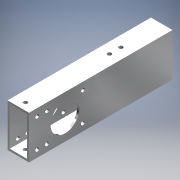
# Autodesk Inventor part: SupportExtrusion
Saved by Autodesk Inventor 2019.4 (Build 234330000, 330)
## iProperties
Created: 2019-12-31
Part Number: SupportExtrusion
Material: Aluminum 6061
Document SubType Name: Modeling
Designer: Mark
Mass: 206.469 g
Surface Area: 554.94 cm^2
Volume: 76.4699 cm^3
Density: 2.7 g/cm^3
Appearance: Aluminum - Flat
Author: Mark
Autodesk Inventor part; units mm, degrees
ref_plane "YZ Plane" through (0, 0, 0) normal (1, 0, 0) x (0, 1, 0)
ref_plane "XZ Plane" through (0, 0, 0) normal (0, 1, 0) x (-1, 0, 0)
ref_plane "XY Plane" through (0, 0, 0) normal (0, 0, 1) x (1, 0, 0)
sketch "Sketch1" plane through (0, 0, 0) normal (0, 0, 1) x (1, 0, 0)
  line L0 (-15, -30) -> (15, -30)
  line L1 (15, -30) -> (15, 30)
  line L2 (15, 30) -> (-15, 30)
  line L3 (-15, 30) -> (-15, -30)
  line L4 (-15, -30) -> (15, 30) construction
  line L5 (15, -30) -> (-15, 30) construction
  line L6 (-12, -27) -> (12, -27)
  line L7 (12, -27) -> (12, 27)
  line L8 (12, 27) -> (-12, 27)
  line L9 (-12, 27) -> (-12, -27)
  line L10 (-12, -27) -> (12, 27) construction
  line L11 (12, -27) -> (-12, 27) construction
  point P0 (0, 0)
  dimension "d0" = 30
  dimension "d1" = 60
  dimension "d2" = 24
  dimension "d3" = 54
  constraints: 24 end point, 4 midpoint, 4 parallel, 2 horizontal, 2 perpendicular
  measures "d0" distance of L2.end L1.end
  measures "d1" distance of L1.end L0.end
  measures "d2" distance of L8.end L7.end
  measures "d3" distance of L7.end L6.end
extrude "Extrusion1" add sketch "Sketch1" along normal blind 200
sketch "Sketch2" plane through (-15, -30, 0) normal (-1, 0, 0) x (0, 0, 1)
  circle A0 centre (188.5, 50) radius 2.75
  circle A1 centre (188.5, 10) radius 2.75
  line L0 (200, 60) -> (200, 0) projected
  line L1 (0, 0) -> (200, 0) projected
  line L2 (0, 60) -> (200, 60) projected
  point P0 (0, 30)
  dimension "d6" = 5.5
  dimension "d7" = 5.5
  dimension "d8" = 11.5
  dimension "d9" = 10
  dimension "d10" = 11.5
  dimension "d11" = 10
  constraints: 2 centre point
  measures "d6" diameter of A0
  measures "d7" diameter of A1
  measures "d8" distance from line of L0 A1.centre
  measures "d9" distance from line of L1 A1.centre
  measures "d10" distance from line of L0 A0.centre
  measures "d11" distance from line of L2 A0.centre
extrude "Extrusion2" cut sketch "Sketch2" against normal blind 30
sketch "Sketch3" plane through (-15, 30, 0) normal (0, 1, 0) x (1, 0, 0)
  circle A0 centre (15, -73) radius 2.75
  circle A1 centre (15, -57) radius 2.75
  line L0 (0, 0) -> (0, -200) projected
  line L1 (30, -200) -> (0, -200) projected
  circle A2 centre (15, -190) radius 2.75
  line L2 (30, 0) -> (30, -200) projected
  point P0 (15, 0)
  dimension "d14" = 5.5
  dimension "d15" = 5.5
  dimension "d16" = 15
  dimension "d17" = 15
  dimension "d18" = 127
  dimension "d19" = 16
  dimension "d40" = 5.5
  dimension "d41" = 10
  dimension "d42" = 15
  constraints: 3 centre point
  measures "d14" diameter of A0
  measures "d15" diameter of A1
  measures "d16" distance from line of L0 A1.centre
  measures "d17" distance from line of L0 A0.centre
  measures "d18" distance from line of L1 A0.centre
  measures "d19" distance of A0.centre A1.centre
  measures "d40" diameter of A2
  measures "d41" distance from line of L1 A2.centre
  measures "d42" distance from line of L2 A2.centre
extrude "Extrusion3" cut sketch "Sketch3" against normal blind 60
sketch "Sketch4" plane through (-15, -30, 0) normal (-1, 0, 0) x (0, 0, 1)
  circle A0 centre (150, 30) radius 20
  line L0 (125, 50) -> (175, 50)
  line L1 (175, 50) -> (175, 10)
  line L2 (175, 10) -> (125, 10)
  line L3 (125, 10) -> (125, 50)
  line L4 (125, 50) -> (175, 10) construction
  line L5 (175, 50) -> (125, 10) construction
  circle A1 centre (175, 50) radius 2.75
  circle A2 centre (175, 10) radius 2.75
  circle A3 centre (125, 10) radius 2.75
  circle A4 centre (125, 50) radius 2.75
  line L6 (200, 60) -> (200, 0) projected
  line L7 (0, 0) -> (200, 0) projected
  circle A5 centre (75, 50) radius 2.75
  circle A6 centre (100, 30) radius 20
  circle A7 centre (125, 50) radius 2.75
  circle A8 centre (125, 10) radius 2.75
  circle A9 centre (75, 10) radius 2.75
  circle A10 centre (25, 50) radius 2.75
  circle A11 centre (50, 30) radius 20
  circle A12 centre (75, 50) radius 2.75
  circle A13 centre (75, 10) radius 2.75
  circle A14 centre (25, 10) radius 2.75
  circle A15 centre (-25, 50) radius 2.75
  circle A16 centre (0, 30) radius 20
  circle A17 centre (25, 50) radius 2.75
  circle A18 centre (25, 10) radius 2.75
  circle A19 centre (-25, 10) radius 2.75
  circle A20 centre (-75, 50) radius 2.75
  circle A21 centre (-50, 30) radius 20
  circle A22 centre (-25, 50) radius 2.75
  circle A23 centre (-25, 10) radius 2.75
  circle A24 centre (-75, 10) radius 2.75
  circle A25 centre (-125, 50) radius 2.75
  circle A26 centre (-100, 30) radius 20
  circle A27 centre (-75, 50) radius 2.75
  circle A28 centre (-75, 10) radius 2.75
  circle A29 centre (-125, 10) radius 2.75
  circle A30 centre (-175, 50) radius 2.75
  circle A31 centre (-150, 30) radius 20
  circle A32 centre (-125, 50) radius 2.75
  circle A33 centre (-125, 10) radius 2.75
  circle A34 centre (-175, 10) radius 2.75
  circle A35 centre (-225, 50) radius 2.75
  circle A36 centre (-200, 30) radius 20
  circle A37 centre (-175, 50) radius 2.75
  circle A38 centre (-175, 10) radius 2.75
  circle A39 centre (-225, 10) radius 2.75
  circle A40 centre (-275, 50) radius 2.75
  circle A41 centre (-250, 30) radius 20
  circle A42 centre (-225, 50) radius 2.75
  circle A43 centre (-225, 10) radius 2.75
  circle A44 centre (-275, 10) radius 2.75
  circle A45 centre (-325, 50) radius 2.75
  circle A46 centre (-300, 30) radius 20
  circle A47 centre (-275, 50) radius 2.75
  circle A48 centre (-275, 10) radius 2.75
  circle A49 centre (-325, 10) radius 2.75
  point P0 (0, 30)
  dimension "d22" = 40
  dimension "d23" = 50
  dimension "d24" = 40
  dimension "d25" = 5.5
  dimension "d26" = 5.5
  dimension "d27" = 5.5
  dimension "d28" = 5.5
  dimension "d29" = 50
  dimension "d30" = 10
  dimension "d33" = 50
  constraints: 50 centre point, 12 end point, 4 coincident, 2 horizontal, 2 midpoint, 2 parallel, 1 perpendicular, 90 other
  measures "d22" diameter of A0
  measures "d23" distance of L1.end L2.end
  measures "d24" distance of L0.end L1.end
  measures "d25" diameter of A1
  measures "d26" diameter of A2
  measures "d27" diameter of A3
  measures "d28" diameter of A4
  measures "d29" distance from line of L6 A0.centre
  measures "d30" distance between parallel lines of L7 L2
  measures "d33" distance of A4.centre A5.centre
extrude "Extrusion4" cut sketch "Sketch4" against normal blind 60 contours A0 | A4 L3 L0 | L0 L3 A4 | A1 L1 L0 | L0 L1 A1 | A2 L1 L2 | L2 L1 A2 | A3 L3 L2 | L2 L3 A3
sketch "Sketch5" plane through (-15, -30, 0) normal (-1, 0, 0) x (0, 0, 1)
  circle A0 centre (38.5, 50) radius 2.75
  circle A1 centre (91.5, 50) radius 2.75
  circle A2 centre (91.5, 10) radius 2.75
  circle A3 centre (38.5, 10) radius 2.75
  line L0 (0, 60) -> (200, 60) projected
  line L1 (0, 60) -> (0, 0) projected
  point P0 (0, 30)
  dimension "d43" = 5.5
  dimension "d44" = 5.5
  dimension "d45" = 5.5
  dimension "d46" = 5.5
  dimension "d47" = 40
  dimension "d48" = 40
  dimension "d49" = 40
  dimension "d50" = 53
  dimension "d51" = 53
  dimension "d52" = 10
  dimension "d53" = 53
  dimension "d54" = 38.5
  constraints: 4 centre point
  measures "d43" diameter of A0
  measures "d44" diameter of A1
  measures "d45" diameter of A2
  measures "d46" diameter of A3
  measures "d47" distance of A0.centre A3.centre
  measures "d48" distance of A2.centre A1.centre
  measures "d49" vertical distance of A3.centre A1.centre
  measures "d50" distance of A1.centre A0.centre
  measures "d51" distance of A3.centre A2.centre
  measures "d52" distance from line of L0 A0.centre
  measures "d53" horizontal distance of A2.centre A0.centre
  measures "d54" distance from line of L1 A0.centre
extrude "Extrusion5" cut sketch "Sketch5" against normal blind 60
body "Solid1"
